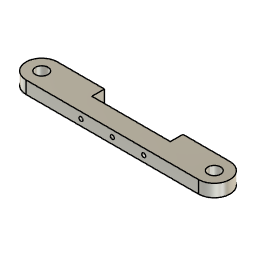
Arm Mount Plate Right (Autodesk Fusion 360 design; units mm, degrees)
Autodesk Fusion 360 part; units mm, degrees
note: some values were not read from the file. Chosen so that the rebuilt part matches the saved one: which bodies a step acts on; how an offset face is resized. Set by a fixed rule: which sketch regions a step uses.
sketch "スケッチ10" plane through (0, 0, 0) normal (0, 0, 1) x (1, 0, 0)
  line L0 (-55, -10) -> (55, -10)
  line L1 (55, -10) -> (55, 10)
  line L2 (55, 10) -> (-55, 10)
  line L3 (-55, 10) -> (-55, -10)
  line L4 (-55, -10) -> (55, 10) construction
  line L5 (55, -10) -> (-55, 10) construction
  circle A0 centre (-55, 0) radius 4.05
  circle A1 centre (55, 0) radius 4.05
  circle A2 centre (-55, 0) radius 10
  circle A3 centre (55, 0) radius 10
  line L6 (-25, -4) -> (25, -4)
  line L7 (25, -4) -> (25, 4)
  line L8 (25, 4) -> (-25, 4)
  line L9 (-25, 4) -> (-25, -4)
  line L10 (-25, -4) -> (25, 4) construction
  line L11 (25, -4) -> (-25, 4) construction
  dimension "d70" = 110
  dimension "d71" = 20
  dimension "d72" = 8.1
  dimension "d73" = 8.1
  dimension "d74" = 50
  dimension "d75" = 8
  constraint horizontal L0
  constraint perpendicular L0 L1
  constraint parallel L0 L2
  constraint parallel L1 L3
  constraint coincident L4 origin
  constraint coincident L5 origin
  constraint midpoint L3 A0.centre
  constraint midpoint L1 A1.centre
  constraint concentric A0 A2
  constraint coincident L0.start A2
  constraint concentric A1 A3
  constraint coincident L0.end A3
  constraint horizontal L6
  constraint perpendicular L6 L7
  constraint parallel L6 L8
  constraint parallel L7 L9
  constraint coincident L10 origin
  constraint coincident L11 origin
  measures "d70" distance of L1.end L2.end
  measures "d71" distance of L0.end L1.end
  measures "d72" diameter of A0
  measures "d73" diameter of A1
  measures "d74" distance of L7.end L8.end
  measures "d75" distance of L6.end L7.end
extrude "押し出し12" add sketch "スケッチ10" along normal blind 8 contours L0 L2 A2 A3 | L3 A0 A2 | L3 A0 A2 | L1 A1 A3 | L1 A1 A3 makes body 1
extrude "押し出し26" cut 1 faces at (-25, 1.3333, 2.6667) along direction (-1, 0, 0) blind 20 on bodies 1 bodies 1
extrude "押し出し27" add 1 faces at (25, -1.3333, 2.6667) along direction (-1, 0, 0) blind 20 on bodies 1 bodies 1
copy_body "ボディのコピーと貼り付け1" bodies 1 makes body 2
move_body "移動1" bodies 2 to x (1, 0, 0) y (0, 1, 0) z (0, 0, 1) at (0, -136, 0)
sketch "スケッチ19" plane through (0, 0, 8) normal (0, 0, 1) x (-1, 0, 0)
  arc A0 (-55, 10) -> (-55, -10) centre (-55, 0) ccw
  line L0 (-55, -10) -> (55, -10)
  arc A1 (55, -10) -> (55, 10) centre (55, 0) ccw
  line L1 (55, 10) -> (-55, 10)
  circle A2 centre (-55, 0) radius 4.05
  circle A3 centre (55, 0) radius 4.05
  line L2 (-5, 4) -> (45, 4)
  line L3 (45, 4) -> (45, -4)
  line L4 (45, -4) -> (-5, -4)
  line L5 (-5, -4) -> (-5, 4)
  line L6 (45, 4) -> (45, 129)
  line L7 (-5, 4) -> (-5, 129)
  line L8 (45, 4) -> (-5, 4)
  line L9 (-5, 129) -> (45, 129)
  dimension "d136" = 125
  dimension "d137" = 125
  constraint coincident L2.end L3.start
  constraint perpendicular L1 L6
  constraint coincident L2.start L5.end
  constraint perpendicular L2 L7
  measures "d136" distance of L2.end L6.end
  measures "d137" distance of L2.start L7.end
extrude "押し出し28" add sketch "スケッチ19" against normal blind 8 contours L1 L6 L7 L9 bodies 1 2
sketch "スケッチ20" plane through (0, 0, 8) normal (0, 0, 1) x (-1, 0, 0)
  circle A0 centre (-55, 136) radius 4.05
  circle A1 centre (55, 136) radius 4.05
  line L0 (-5, 140) -> (45, 140)
  line L1 (45, 140) -> (45, 132)
  line L2 (45, 132) -> (-5, 132)
  line L3 (-5, 132) -> (-5, 140)
  arc A2 (-55, 10) -> (-55, -10) centre (-55, 0) ccw
  line L4 (-55, -10) -> (55, -10)
  arc A3 (55, -10) -> (55, 10) centre (55, 0) ccw
  line L5 (55, 10) -> (45, 10)
  line L6 (45, 10) -> (45, 126)
  line L7 (45, 126) -> (55, 126)
  arc A4 (55, 126) -> (55, 146) centre (55, 136) ccw
  line L8 (55, 146) -> (-55, 146)
  arc A5 (-55, 146) -> (-55, 126) centre (-55, 136) ccw
  line L9 (-55, 126) -> (-5, 126)
  line L10 (-5, 126) -> (-5, 10)
  line L11 (-5, 10) -> (-55, 10)
  circle A6 centre (-55, 0) radius 4.05
  circle A7 centre (55, 0) radius 4.05
  line L12 (-5, 4) -> (45, 4)
  line L13 (45, 4) -> (45, -4)
  line L14 (45, -4) -> (-5, -4)
  line L15 (-5, -4) -> (-5, 4)
  line L16 (-5, 68) -> (0, 68)
  circle A8 centre (0, 68) radius 25
  dimension "d143" = 5
  dimension "d144" = 50
  constraint midpoint L10 L16.start
  constraint perpendicular L10 L16
  constraint coincident L16.end A8.centre
  measures "d143" distance of L16.start L16.end
  measures "d144" diameter of A8
extrude "押し出し29" cut sketch "スケッチ20" against normal blind 8 contours L10 A8 picked at (14.9093, 66.7738) bodies 1
sketch "スケッチ21" plane through (0, 0, 8) normal (0, 0, 1) x (-1, 0, 0)
  arc A0 (-5, 43.5051) -> (-5, 92.4949) centre (0, 68) ccw
  line L0 (-5, 43.5051) -> (-5, 10)
  line L1 (-5, 10) -> (-55, 10)
  arc A1 (-55, 10) -> (-55, -10) centre (-55, 0) ccw
  line L2 (-55, -10) -> (55, -10)
  arc A2 (55, -10) -> (55, 10) centre (55, 0) ccw
  line L3 (55, 10) -> (45, 10)
  line L4 (45, 10) -> (45, 126)
  line L5 (45, 126) -> (55, 126)
  arc A3 (55, 126) -> (55, 146) centre (55, 136) ccw
  line L6 (55, 146) -> (-55, 146)
  arc A4 (-55, 146) -> (-55, 126) centre (-55, 136) ccw
  line L7 (-55, 126) -> (-5, 126)
  line L8 (-5, 126) -> (-5, 92.4949)
  circle A5 centre (-55, 136) radius 4.05
  circle A6 centre (55, 136) radius 4.05
  line L9 (-5, 140) -> (45, 140)
  line L10 (45, 140) -> (45, 132)
  line L11 (45, 132) -> (-5, 132)
  line L12 (-5, 132) -> (-5, 140)
  circle A7 centre (-55, 0) radius 4.05
  circle A8 centre (55, 0) radius 4.05
  line L13 (-5, 4) -> (45, 4)
  line L14 (45, 4) -> (45, -4)
  line L15 (45, -4) -> (-5, -4)
  line L16 (-5, -4) -> (-5, 4)
  line L17 (20, 4) -> (20, 132)
  line L18 (0, 68) -> (0, 93)
  line L19 (0, 68) -> (0, 65.1188)
  line L20 (0, 65.1188) -> (0, 43)
  line L21 (0, 93) -> (20, 93)
  line L22 (0, 43) -> (20, 43)
  line L23 (20, 43) -> (20, 39)
  line L24 (20, 93) -> (20, 97)
  line L25 (-5, 43) -> (45, 43)
  line L26 (45, 43) -> (45, 35)
  line L27 (45, 35) -> (-5, 35)
  line L28 (-5, 35) -> (-5, 43)
  line L29 (-5, 43) -> (45, 35) construction
  line L30 (45, 43) -> (-5, 35) construction
  line L31 (-5, 101) -> (45, 101)
  line L32 (45, 101) -> (45, 93)
  line L33 (45, 93) -> (-5, 93)
  line L34 (-5, 93) -> (-5, 101)
  line L35 (-5, 101) -> (45, 93) construction
  line L36 (45, 101) -> (-5, 93) construction
  point P0 (20, 39)
  point P1 (20, 97)
  dimension "d145" = 4
  dimension "d146" = 4
  dimension "d147" = 8
  dimension "d148" = 8
  constraint midpoint L13 L17.start
  constraint midpoint L11 L17.end
  constraint coincident A0.centre L18.start
  constraint coincident A0 L18.end
  constraint parallel L17 L18
  constraint coincident A0 L20.end
  constraint parallel L18 L20
  constraint coincident L17 L21.end
  constraint tangent A0 L21
  constraint coincident L17 L22.end
  constraint tangent A0 L22
  constraint perpendicular L17 L22
  constraint perpendicular L22 L23
  constraint perpendicular L21 L24
  constraint horizontal L25
  constraint perpendicular L25 L26
  constraint parallel L25 L27
  constraint parallel L26 L28
  constraint coincident L29 P0
  constraint coincident L30 P0
  constraint coincident P0 L23.end
  constraint horizontal L31
  constraint perpendicular L31 L32
  constraint parallel L31 L33
  constraint parallel L32 L34
  constraint coincident L35 P1
  constraint coincident L36 P1
  constraint coincident P1 L24.end
  measures "d145" distance of L22.end P0
  measures "d146" distance of L21.end P1
  measures "d147" distance of L25.end L26.end
  measures "d148" distance of L31.end L32.end
extrude "押し出し30" cut sketch "スケッチ21" against normal blind 8 contours A0 L0 L25 | L0 L17 L22 L23 L25 L27 L28 | L4 L17 L23 L25 L26 L27 | L8 L17 L21 L24 L31 L33 L34 | A0 L8 L33 | L4 L17 L24 L31 L32 L33 bodies 1 makes body 3 at (-11.6667, -117.6667, 0) makes body 4 at (-11.6667, -26.6667, 8)
sketch "スケッチ22" plane through (0, 0, 8) normal (0, 0, 1) x (-1, 0, 0)
  line L0 (-5, 140) -> (45, 140)
  line L1 (45, 140) -> (45, 132)
  line L2 (45, 132) -> (-5, 132)
  line L3 (-5, 132) -> (-5, 140)
  circle A0 centre (55, 136) radius 4.05
  circle A1 centre (-55, 136) radius 4.05
  line L4 (-5, 101) -> (45, 101)
  line L5 (45, 101) -> (45, 126)
  line L6 (45, 126) -> (55, 126)
  arc A2 (55, 126) -> (55, 146) centre (55, 136) ccw
  line L7 (55, 146) -> (-55, 146)
  arc A3 (-55, 146) -> (-55, 126) centre (-55, 136) ccw
  line L8 (-55, 126) -> (-5, 126)
  line L9 (-5, 126) -> (-5, 101)
  line L10 (45, 140) -> (45, 146)
  line L11 (-5, 140) -> (-5, 146)
  line L12 (-5, 146) -> (45, 146)
  line L13 (45, 146) -> (45, 154)
  line L14 (45, 154) -> (-5, 154)
  line L15 (-5, 154) -> (-5, 146)
  line L16 (-5, 154) -> (45, 154)
  line L17 (45, 154) -> (45, 160)
  line L18 (45, 160) -> (-5, 160)
  line L19 (-5, 160) -> (-5, 154)
  line L20 (45, 160) -> (51, 160)
  line L21 (51, 160) -> (51, 146)
  line L22 (51, 146) -> (45, 146)
  line L23 (45, 146) -> (45, 160)
  line L24 (-5, 160) -> (-11, 160)
  line L25 (-11, 160) -> (-11, 146)
  line L26 (-11, 146) -> (-5, 146)
  line L27 (-5, 146) -> (-5, 160)
  dimension "d151" = 8
  dimension "d152" = 6
  dimension "d153" = 6
  dimension "d154" = 6
  constraint coincident L0.end L1.start
  constraint coincident L7 L10.end
  constraint perpendicular L7 L10
  constraint coincident L0.start L3.end
  constraint coincident L7 L11.end
  constraint perpendicular L7 L11
  constraint horizontal L12
  constraint vertical L13
  constraint horizontal L14
  constraint vertical L15
  constraint horizontal L16
  constraint vertical L17
  constraint horizontal L18
  constraint vertical L19
  constraint horizontal L20
  constraint vertical L21
  constraint horizontal L22
  constraint vertical L23
  constraint horizontal L24
  constraint vertical L25
  constraint horizontal L26
  constraint vertical L27
  measures "d151" distance of L11.end L14.end
  measures "d152" distance of L14.end L18.end
  measures "d153" distance of L17.end L20.end
  measures "d154" distance of L18.end L24.end
extrude "押し出し31" add sketch "スケッチ22" against normal blind 8 contours L0 L1 L2 L3 | L7 L15 L19 L24 L25 L26 L27 | L7 L13 L17 L20 L21 L22 L23 | L14 L16 L17 L18 L19 L23 L27 bodies 3
sketch "スケッチ23" plane through (0, 0, 8) normal (0, 0, 1) x (-1, 0, 0)
  line L0 (-5, 4) -> (45, 4)
  line L1 (45, 4) -> (45, -4)
  line L2 (45, -4) -> (-5, -4)
  line L3 (-5, -4) -> (-5, 4)
  circle A0 centre (55, 0) radius 4.05
  circle A1 centre (-55, 0) radius 4.05
  line L4 (45, 35) -> (-5, 35)
  line L5 (-5, 35) -> (-5, 10)
  line L6 (-5, 10) -> (-55, 10)
  arc A2 (-55, 10) -> (-55, -10) centre (-55, 0) ccw
  line L7 (-55, -10) -> (55, -10)
  arc A3 (55, -10) -> (55, 10) centre (55, 0) ccw
  line L8 (55, 10) -> (45, 10)
  line L9 (45, 10) -> (45, 35)
  line L10 (45, -4) -> (45, -10)
  line L11 (-5, -4) -> (-5, -10)
  line L12 (45, -10) -> (-5, -10)
  line L13 (-5, -10) -> (-5, -18)
  line L14 (-5, -18) -> (45, -18)
  line L15 (45, -18) -> (45, -10)
  line L16 (45, -18) -> (-5, -18)
  line L17 (-5, -18) -> (-5, -24)
  line L18 (-5, -24) -> (45, -24)
  line L19 (45, -24) -> (45, -18)
  line L20 (45, -24) -> (51, -24)
  line L21 (51, -24) -> (51, -10)
  line L22 (51, -10) -> (45, -10)
  line L23 (45, -10) -> (45, -24)
  line L24 (-5, -24) -> (-11, -24)
  line L25 (-11, -24) -> (-11, -10)
  line L26 (-11, -10) -> (-5, -10)
  line L27 (-5, -10) -> (-5, -24)
  dimension "d157" = 8
  dimension "d158" = 6
  dimension "d159" = 6
  dimension "d160" = 6
  constraint coincident L1.end L2.start
  constraint coincident L7 L10.end
  constraint perpendicular L7 L10
  constraint coincident L2.end L3.start
  constraint coincident L7 L11.end
  constraint perpendicular L7 L11
  constraint horizontal L12
  constraint vertical L13
  constraint horizontal L14
  constraint vertical L15
  constraint horizontal L16
  constraint vertical L17
  constraint horizontal L18
  constraint vertical L19
  constraint horizontal L20
  constraint vertical L21
  constraint horizontal L22
  constraint vertical L23
  constraint horizontal L24
  constraint vertical L25
  constraint horizontal L26
  constraint vertical L27
  measures "d157" distance of L10.end L14.end
  measures "d158" distance of L14.end L18.end
  measures "d159" distance of L18.end L20.end
  measures "d160" distance of L17.end L24.end
extrude "押し出し32" add sketch "スケッチ23" against normal blind 8 contours L0 L1 L2 L3 | L7 L13 L17 L24 L25 L26 L27 | L7 L15 L19 L20 L21 L22 L23 | L14 L16 L17 L18 L19 L23 L27 bodies 4
sketch "スケッチ24" plane through (0, -10, 0) normal (0, -1, 0) x (1, 0, 0)
  line L0 (-45, 0) -> (-45, 8)
  line L1 (-45, 8) -> (-55, 8)
  line L2 (-55, 8) -> (-55, 0)
  line L3 (-55, 0) -> (-45, 0)
  line L4 (-45, 0) -> (-51, 0)
  line L5 (-51, 0) -> (-51, 8)
  line L6 (-51, 8) -> (-45, 8)
  line L7 (-45, 8) -> (-45, 0)
  dimension "d163" = 6
  constraint horizontal L4
  constraint vertical L5
  constraint horizontal L6
  constraint vertical L7
  constraint coincident L0.start L3.end
  measures "d163" distance of L0.start L4.end
extrude "押し出し33" add sketch "スケッチ24" along normal blind 117 contours L0 L1 L3 L4 L5 L6 L7 bodies 1 3 4
split "分割1" by plane through (55, -126, 0) normal (0, 1, 0) bodies 1 makes body 5 at (-30.3333, -18.3333, 0)
delete_body "RemoveBody1" bodies 5
sketch "スケッチ26" plane through (0, -126, 0) normal (0, 1, 0) x (-1, 0, 0)
  line L0 (-55, 0) -> (55, 0)
  line L1 (55, 0) -> (55, 8)
  line L2 (55, 8) -> (-55, 8)
  line L3 (-55, 8) -> (-55, 0)
  line L4 (0, 0) -> (0, 8)
  line L5 (30, 0) -> (-30, 0)
  line L6 (-30, 0) -> (-30, 8)
  line L7 (-30, 8) -> (30, 8)
  line L8 (30, 8) -> (30, 0)
  line L9 (30, 0) -> (-30, 8) construction
  line L10 (-30, 0) -> (30, 8) construction
  point P0 (0, 4)
  dimension "d169" = 60
  dimension "d170" = 8
  constraint coincident L4.start origin
  constraint midpoint L2 L4.end
  constraint horizontal L5
  constraint perpendicular L5 L6
  constraint parallel L5 L7
  constraint parallel L6 L8
  constraint coincident L9 P0
  constraint coincident L10 P0
  constraint midpoint L4 P0
  measures "d169" distance of L6.end L7.end
  measures "d170" distance of L5.end L6.end
extrude "押し出し35" add sketch "スケッチ26" along normal blind 40 contours L0 L2 L4 L5 L6 L7 | L0 L2 L4 L5 L7 L8 bodies 1
sketch "スケッチ27" plane through (0, -86, 0) normal (0, 1, 0) x (-1, 0, 0)
  line L0 (30, 8) -> (-30, 8)
  line L1 (-30, 8) -> (-30, 0)
  line L2 (-30, 0) -> (30, 0)
  line L3 (30, 0) -> (30, 8)
  line L4 (-30, 8) -> (-25, 8)
  line L5 (-25, 8) -> (-25, 0)
  line L6 (-25, 0) -> (-30, 0)
  line L7 (-30, 0) -> (-30, 8)
  line L8 (30, 8) -> (25, 8)
  line L9 (25, 8) -> (25, 0)
  line L10 (25, 0) -> (30, 0)
  line L11 (30, 0) -> (30, 8)
  dimension "d173" = 5
  dimension "d174" = 8
  dimension "d175" = 5
  dimension "d176" = 8
  constraint horizontal L4
  constraint vertical L5
  constraint horizontal L6
  constraint vertical L7
  constraint coincident L0.end L1.start
  constraint horizontal L8
  constraint vertical L9
  constraint horizontal L10
  constraint vertical L11
  constraint coincident L0.start L3.end
  measures "d173" distance of L0.end L4.end
  measures "d174" distance of L0.end L1.end
  measures "d175" distance of L0.start L8.end
  measures "d176" distance of L0.start L2.end
extrude "押し出し36" add sketch "スケッチ27" along normal blind 8 contours L0 L2 L3 L8 L9 L10 L11 | L0 L1 L2 L4 L5 L6 L7 bodies 1
split "分割2" by plane through (-55, -146, 0) normal (0, -1, 0) bodies 1 makes body 6 at (-30.3333, -160, 5.3333)
delete_body "RemoveBody2" bodies 6
sketch "スケッチ28" plane through (0, -146, 0) normal (0, -1, 0) x (1, 0, 0)
  line L0 (55, 8) -> (-55, 8)
  line L1 (-55, 8) -> (-55, 0)
  line L2 (-55, 0) -> (55, 0)
  line L3 (55, 0) -> (55, 8)
  line L4 (0, 0) -> (0, 8)
  line L5 (30, 0) -> (-30, 0)
  line L6 (-30, 0) -> (-30, 8)
  line L7 (-30, 8) -> (30, 8)
  line L8 (30, 8) -> (30, 0)
  line L9 (30, 0) -> (-30, 8) construction
  line L10 (-30, 0) -> (30, 8) construction
  line L11 (-30, 8) -> (-25, 8)
  line L12 (-25, 8) -> (-25, 0)
  line L13 (-25, 0) -> (-30, 0)
  line L14 (-30, 0) -> (-30, 8)
  line L15 (30, 8) -> (25, 8)
  line L16 (25, 8) -> (25, 0)
  line L17 (25, 0) -> (30, 0)
  line L18 (30, 0) -> (30, 8)
  point P0 (0, 4)
  dimension "d179" = 60
  dimension "d180" = 8
  dimension "d181" = 5
  dimension "d182" = 8
  dimension "d183" = 5
  dimension "d184" = 8
  constraint coincident L4.start origin
  constraint midpoint L0 L4.end
  constraint horizontal L5
  constraint perpendicular L5 L6
  constraint parallel L5 L7
  constraint parallel L6 L8
  constraint coincident L9 P0
  constraint coincident L10 P0
  constraint midpoint L4 P0
  constraint horizontal L11
  constraint vertical L12
  constraint horizontal L13
  constraint vertical L14
  constraint horizontal L15
  constraint vertical L16
  constraint horizontal L17
  constraint vertical L18
  measures "d179" distance of L6.end L7.end
  measures "d180" distance of L5.end L6.end
  measures "d181" distance of L6.end L11.end
  measures "d182" distance of L6.end L5.end
  measures "d183" distance of L7.end L15.end
  measures "d184" distance of L7.end L5.start
extrude "押し出し37" add sketch "スケッチ28" along normal blind 13 contours L0 L2 L5 L7 L8 L15 L16 L17 L18 | L0 L2 L4 L5 L7 L16 | L0 L2 L4 L5 L7 L12 | L0 L2 L5 L6 L7 L11 L12 L13 L14 bodies 1
extrude "押し出し38" cut sketch "スケッチ28" along normal blind 8 contours L0 L2 L4 L5 L7 L16 | L0 L2 L4 L5 L7 L12 bodies 1
split "分割3" by plane through (55, -126, 0) normal (0, 1, 0) bodies 1 makes body 7 at (8.3333, -112.6667, 8)
delete_body "RemoveBody3" bodies 7
extrude "押し出し39" cut 1 faces at (-8.3333, -146, 5.3333) along direction (0, 1, 0) blind 10 on bodies 1 bodies 1
extrude "押し出し40" add 1 faces at (-8.3333, -154, 5.3333) along direction (0, 1, 0) blind 10 on bodies 1 bodies 1
extrude "押し出し41" cut 1 faces at (-10, -159, 5.3333) along direction (0, 1, 0) blind 10 on bodies 1 bodies 1
extrude "押し出し42" cut 1 faces at (-8.3333, -136, 5.3333) along direction (0, 1, 0) blind 5 on bodies 1 bodies 1
extrude "押し出し43" add 1 faces at (-8.3333, -144, 5.3333) along direction (0, 1, 0) blind 5 on bodies 1 bodies 1
extrude "押し出し44" cut 1 faces at (-10, -149, 5.3333) along direction (0, 1, 0) blind 3 on bodies 1 bodies 1
extrude "押し出し45" cut 1 faces at (-8.3333, -131, 5.3333) along direction (0, 1, 0) blind 5 on bodies 1 bodies 1
extrude "押し出し46" add 1 faces at (-8.3333, -139, 5.3333) along direction (0, 1, 0) blind 5 on bodies 1 bodies 1
sketch "スケッチ29" plane through (0, -134, 0) normal (0, 1, 0) x (-1, 0, 0)
  line L0 (25, 0) -> (25, 8)
  line L1 (25, 8) -> (-25, 8)
  line L2 (-25, 8) -> (-25, 0)
  line L3 (-25, 0) -> (25, 0)
  line L4 (0, 0) -> (0, 8)
  line L5 (0, 4) -> (-20, 4)
  line L6 (0, 4) -> (20, 4)
  circle A0 centre (0, 4) radius 1.25
  circle A1 centre (-20, 4) radius 1.25
  circle A2 centre (20, 4) radius 1.25
  dimension "d205" = 2.5
  dimension "d206" = 2.5
  dimension "d207" = 2.5
  constraint coincident L4.start origin
  constraint midpoint L1 L4.end
  constraint midpoint L4 L5.start
  constraint perpendicular L2 L5
  constraint perpendicular L4 L6
  constraint coincident L5.start L6.start
  constraint coincident L5.end A1.centre
  constraint coincident L6.end A2.centre
  measures "d205" diameter of A0
  measures "d206" diameter of A1
  measures "d207" diameter of A2
extrude "押し出し47" cut sketch "スケッチ29" against normal blind 12 contours L4 L5 A0 | L4 L6 A0 | L4 L6 A0 | L4 L5 A0 | A1 | A2 bodies 1
thread "ねじ1" "ISO Metric profile 3.0 M3x0.5 6H" major diameter 3.086 minor diameter 2.529 pitch 0.5 angle 60 resizes the face on face at (-21.2438, -138, 4.1245) on bodies 1
thread "ねじ2" "ISO Metric profile 3.0 M3x0.5 6H" major diameter 3.086 minor diameter 2.529 pitch 0.5 angle 60 resizes the face on face at (-1.2438, -138, 3.8755) on bodies 1
thread "ねじ3" "ISO Metric profile 3.0 M3x0.5 6H" major diameter 3.086 minor diameter 2.529 pitch 0.5 angle 60 resizes the face on face at (18.7562, -138, 3.8755) on bodies 1
